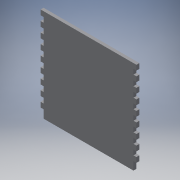
# Autodesk Inventor part: верх
Saved by Autodesk Inventor 2019 (Build 230136000, 136)
## iProperties
Created: 2022-02-24
Part Number: верх
Material: Типовые
Document SubType Name: Modeling
Designer: korsh
Density: 1 g/cm^3
Appearance: По умолчанию
Author: korsh
Autodesk Inventor part; units mm, degrees
ref_plane "YZ Plane" through (0, 0, 0) normal (1, 0, 0) x (0, 1, 0)
ref_plane "XZ Plane" through (0, 0, 0) normal (0, 1, 0) x (-1, 0, 0)
ref_plane "XY Plane" through (0, 0, 0) normal (0, 0, 1) x (1, 0, 0)
sketch "Эскиз1" plane through (0, 0, 0) normal (0, 0, 1) x (1, 0, 0)
  line L0 (0, 20) -> (0, 30) projected
  line L1 (0, 20) -> (6, 20) projected
  line L2 (6, 30) -> (6, 20) projected
  line L3 (0, 30) -> (6, 30) projected
  line L4 (0, 0) -> (0, 10) projected
  line L5 (0, 0) -> (6, 0) projected
  line L6 (6, 10) -> (6, 0) projected
  line L7 (0, 10) -> (6, 10) projected
  line L8 (0, -20) -> (0, -10) projected
  line L9 (0, -20) -> (6, -20) projected
  line L10 (6, -10) -> (6, -20) projected
  line L11 (0, -10) -> (6, -10) projected
  line L12 (0, -40) -> (0, -30) projected
  line L13 (0, -40) -> (6, -40) projected
  line L14 (6, -30) -> (6, -40) projected
  line L15 (0, -30) -> (6, -30) projected
  line L16 (0, -60) -> (0, -50) projected
  line L17 (0, -60) -> (6, -60) projected
  line L18 (6, -50) -> (6, -60) projected
  line L19 (0, -50) -> (6, -50) projected
  line L20 (0, -80) -> (0, -70) projected
  line L21 (0, -80) -> (6, -80) projected
  line L22 (6, -70) -> (6, -80) projected
  line L23 (0, -70) -> (6, -70) projected
  line L24 (0, -100) -> (0, -90) projected
  line L25 (0, -100) -> (6, -100) projected
  line L26 (6, -90) -> (6, -100) projected
  line L27 (0, -90) -> (6, -90) projected
  line L28 (0, -120) -> (0, -110) projected
  line L29 (0, -120) -> (6, -120) projected
  line L30 (6, -110) -> (6, -120) projected
  line L31 (0, -110) -> (6, -110) projected
  line L32 (0, -140) -> (0, -130) projected
  line L33 (0, -140) -> (6, -140) projected
  line L34 (6, -130) -> (6, -140) projected
  line L35 (0, -130) -> (6, -130) projected
  line L36 (0, -156.3478) -> (0, -140) projected
  line L37 (-180, -140) -> (-180, -156.3478) projected
  line L38 (-186, -140) -> (-186, -130) projected
  line L39 (-186, -140) -> (-180, -140) projected
  line L40 (-180, -130) -> (-180, -140) projected
  line L41 (-186, -130) -> (-180, -130) projected
  line L42 (-186, -120) -> (-186, -110) projected
  line L43 (-186, -120) -> (-180, -120) projected
  line L44 (-180, -110) -> (-180, -120) projected
  line L45 (-186, -110) -> (-180, -110) projected
  line L46 (-186, -100) -> (-186, -90) projected
  line L47 (-186, -100) -> (-180, -100) projected
  line L48 (-180, -90) -> (-180, -100) projected
  line L49 (-186, -90) -> (-180, -90) projected
  line L50 (-186, -80) -> (-186, -70) projected
  line L51 (-186, -80) -> (-180, -80) projected
  line L52 (-180, -70) -> (-180, -80) projected
  line L53 (-186, -70) -> (-180, -70) projected
  line L54 (-186, -60) -> (-186, -50) projected
  line L55 (-186, -60) -> (-180, -60) projected
  line L56 (-180, -50) -> (-180, -60) projected
  line L57 (-186, -50) -> (-180, -50) projected
  line L58 (-186, -40) -> (-186, -30) projected
  line L59 (-186, -40) -> (-180, -40) projected
  line L60 (-180, -30) -> (-180, -40) projected
  line L61 (-186, -30) -> (-180, -30) projected
  line L62 (-186, 20) -> (-186, 30) projected
  line L63 (-186, 20) -> (-180, 20) projected
  line L64 (-180, 30) -> (-180, 20) projected
  line L65 (-186, 30) -> (-180, 30) projected
  line L66 (-186, 0) -> (-186, 10) projected
  line L67 (-186, 0) -> (-180, 0) projected
  line L68 (-180, 10) -> (-180, 0) projected
  line L69 (-186, 10) -> (-180, 10) projected
  line L70 (-186, -20) -> (-186, -10) projected
  line L71 (-186, -20) -> (-180, -20) projected
  line L72 (-180, -10) -> (-180, -20) projected
  line L73 (-186, -10) -> (-180, -10) projected
  line L74 (0, -156.3478) -> (-180, -156.3478)
  line L75 (-180, -156.3478) -> (-180, 30)
  line L76 (-180, 30) -> (0, 30)
  line L77 (0, 30) -> (0, -156.3478)
  constraints: 8 end point, 2 parallel, 1 horizontal, 1 perpendicular
extrude "Выдавливание1" add sketch "Эскиз1" along normal blind 6
sketch "Эскиз2" plane through (0, 0, 6) normal (0, 0, 1) x (1, 0, 0)
  line L0 (-15, 15) -> (-165, 15)
  line L1 (-165, 15) -> (-165, -141.3478)
  line L2 (-165, -141.3478) -> (-15, -141.3478)
  line L3 (-15, -141.3478) -> (-15, 15)
  line L4 (-186, 10) -> (-186, 0) projected
  line L5 (-186, 0) -> (-180, 0) projected
  line L6 (-180, 0) -> (-180, -10) projected
  line L7 (-180, -10) -> (-186, -10) projected
  line L8 (-186, -10) -> (-186, -20) projected
  line L9 (-186, -20) -> (-180, -20) projected
  line L10 (-180, -20) -> (-180, -30) projected
  line L11 (-180, -30) -> (-186, -30) projected
  line L12 (-186, -30) -> (-186, -40) projected
  line L13 (-186, -40) -> (-180, -40) projected
  line L14 (-180, -40) -> (-180, -50) projected
  line L15 (-180, -50) -> (-186, -50) projected
  line L16 (-186, -50) -> (-186, -60) projected
  line L17 (-186, -60) -> (-180, -60) projected
  line L18 (-180, -60) -> (-180, -70) projected
  line L19 (-180, -70) -> (-186, -70) projected
  line L20 (-186, -70) -> (-186, -80) projected
  line L21 (-186, -80) -> (-180, -80) projected
  line L22 (-180, -80) -> (-180, -90) projected
  line L23 (-180, -90) -> (-186, -90) projected
  line L24 (-186, -90) -> (-186, -100) projected
  line L25 (-186, -100) -> (-180, -100) projected
  line L26 (-180, -100) -> (-180, -110) projected
  line L27 (-180, -110) -> (-186, -110) projected
  line L28 (-186, -110) -> (-186, -120) projected
  line L29 (-186, -120) -> (-180, -120) projected
  line L30 (-180, -120) -> (-180, -130) projected
  line L31 (-180, -130) -> (-186, -130) projected
  line L32 (-186, -130) -> (-186, -140) projected
  line L33 (-186, -140) -> (-180, -140) projected
  line L34 (-180, -140) -> (-180, -156.3478) projected
  line L35 (-180, -156.3478) -> (0, -156.3478) projected
  line L36 (0, -156.3478) -> (0, -140) projected
  line L37 (0, -140) -> (6, -140) projected
  line L38 (6, -140) -> (6, -130) projected
  line L39 (6, -130) -> (0, -130) projected
  line L40 (0, -130) -> (0, -120) projected
  line L41 (0, -120) -> (6, -120) projected
  line L42 (6, -120) -> (6, -110) projected
  line L43 (6, -110) -> (0, -110) projected
  line L44 (0, -110) -> (0, -100) projected
  line L45 (0, -100) -> (6, -100) projected
  line L46 (6, -100) -> (6, -90) projected
  line L47 (6, -90) -> (0, -90) projected
  line L48 (0, -90) -> (0, -80) projected
  line L49 (0, -80) -> (6, -80) projected
  line L50 (6, -80) -> (6, -70) projected
  line L51 (6, -70) -> (0, -70) projected
  line L52 (0, -70) -> (0, -60) projected
  line L53 (0, -60) -> (6, -60) projected
  line L54 (6, -60) -> (6, -50) projected
  line L55 (6, -50) -> (0, -50) projected
  line L56 (0, -50) -> (0, -40) projected
  line L57 (0, -40) -> (6, -40) projected
  line L58 (6, -40) -> (6, -30) projected
  line L59 (6, -30) -> (0, -30) projected
  line L60 (0, -30) -> (0, -20) projected
  line L61 (0, -20) -> (6, -20) projected
  line L62 (6, -20) -> (6, -10) projected
  line L63 (6, -10) -> (0, -10) projected
  line L64 (0, -10) -> (0, 0) projected
  line L65 (0, 0) -> (6, 0) projected
  line L66 (6, 0) -> (6, 10) projected
  line L67 (6, 10) -> (0, 10) projected
  line L68 (0, 10) -> (0, 20) projected
  line L69 (0, 20) -> (6, 20) projected
  line L70 (6, 20) -> (6, 30) projected
  line L71 (6, 30) -> (-186, 30) projected
  line L72 (-186, 30) -> (-186, 20) projected
  line L73 (-186, 20) -> (-180, 20) projected
  line L74 (-180, 20) -> (-180, 10) projected
  line L75 (-180, 10) -> (-186, 10) projected
  dimension "d2" = 15
  dimension "d3" = 15
  dimension "d4" = 15
  dimension "d5" = 15
  constraints: 8 end point, 2 parallel, 1 horizontal, 1 perpendicular
  measures "d2" distance between parallel lines of L0 L71
  measures "d3" distance between parallel lines of L2 L35
  measures "d4" distance between parallel lines of L3 L48
  measures "d5" distance between parallel lines of L1 L18
extrude "Выдавливание2" cut sketch "Эскиз2" against normal blind 6 contours L3 L2 L1 L0
